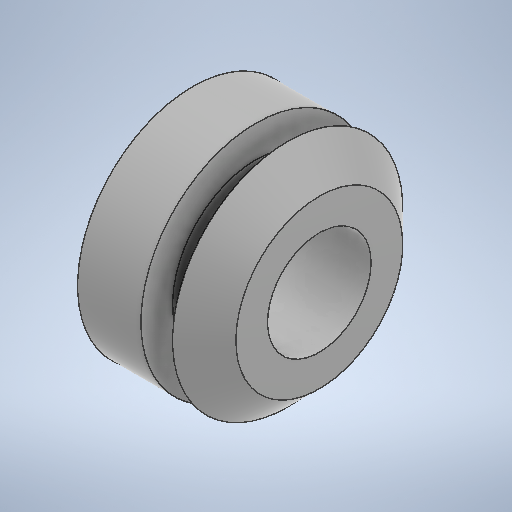
# Autodesk Inventor part: spacer_Φ3.2_1
Saved by Autodesk Inventor 2025 (Build 290162000, 162)
## iProperties
Created: 2025-09-16
Part Number: spacer_Φ3.2_1
Material: 一般
Document SubType Name: Modeling
Designer: sooo1
Density: 1 g/cm^3
Appearance: 滑らか - 標準の灰色
Author: sooo1
Autodesk Inventor part; units mm, degrees
ref_plane "YZ Plane" through (0, 0, 0) normal (1, 0, 0) x (0, 1, 0)
ref_plane "XZ Plane" through (0, 0, 0) normal (0, 1, 0) x (-1, 0, 0)
sketch "スケッチ1" plane through (0, 0, 0) normal (1, 0, 0) x (0, 1, 0)
  circle A0 centre (0, 0) radius 3.635
  circle A1 centre (0, 0) radius 1.635
  circle A2 centre (0, 0) radius 2.635
  dimension "d0" = 3.27
  dimension "d1" = 2
  dimension "d7" = 1
  constraints: 3 centre point, 3 coincident
  measures "d0" diameter of A1
  measures "d1" radial gap between concentric circles of A1 A0
  measures "d7" radial gap between concentric circles of A0 A2
extrude "押し出し1" add sketch "スケッチ1" along normal mid plane 4 contours A0 | A2
ref_plane "作業平面1" through (1, 0, 0) normal (1, 0, 0) x (0, 0, -1)
extrude "押し出し3" cut sketch "スケッチ1" against normal blind 1 from surface at 1 contours A0
chamfer "面取り3" distance 1 angle 45 1 edges at (2, -3.635, 0)
